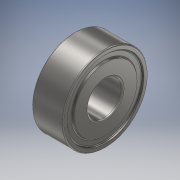
# Autodesk Inventor part: Rear Compression Bearing
Saved by Autodesk Inventor 2019 (Build 230136000, 136)
## iProperties
Created: 2017-03-14
Part Number: Rear Compression Bearing
Material: Stainless Steel
Document SubType Name: Modeling
Designer: zhangxun
Density: 8 g/cm^3
Appearance: Semi-Polished
Author: zhangxun
Autodesk Inventor part; units mm, degrees
ref_plane "YZ Plane" through (0, 0, 0) normal (1, 0, 0) x (0, 1, 0)
ref_plane "XZ Plane" through (0, 0, 0) normal (0, 1, 0) x (-1, 0, 0)
ref_plane "XY Plane" through (0, 0, 0) normal (0, 0, 1) x (1, 0, 0)
sketch "Sketch1" plane through (0, 0, 0) normal (0, 1, 0) x (-1, 0, 0)
  line L0 (19.5, 11) -> (1.5, 11)
  arc A0 (0.5, 12) -> (1.5, 11) centre (1.5, 12) ccw
  line L1 (0.5, 12) -> (0.5, 20.35)
  line L2 (0.5, 20.35) -> (2.3602, 20.35)
  arc A1 (1.5, 21.2102) -> (2.3602, 20.35) centre (2.3602, 21.2102) ccw
  line L3 (1.5, 21.2102) -> (1.5, 23.7908)
  arc A2 (2.3187, 24.65) -> (1.5, 23.7908) centre (2.3602, 23.7908) ccw
  line L4 (2.3187, 24.65) -> (1.5, 24.65)
  line L5 (1.5, 24.65) -> (1.5, 24.7964)
  line L6 (1.5, 24.7964) -> (0.5, 24.7964)
  line L7 (0.5, 24.7964) -> (0.5, 26.9)
  arc A3 (1.1, 27.5) -> (0.5, 26.9) centre (1.1, 26.9) ccw
  line L8 (1.1, 27.5) -> (19.9, 27.5)
  arc A4 (20.5, 26.9) -> (19.9, 27.5) centre (19.9, 26.9) ccw
  line L9 (20.5, 26.9) -> (20.5, 24.8239)
  line L10 (20.5, 24.8239) -> (19.5, 24.8239)
  line L11 (19.5, 24.8239) -> (19.5, 24.65)
  line L12 (19.5, 24.65) -> (18.6813, 24.65)
  arc A5 (19.5, 23.7908) -> (18.6813, 24.65) centre (18.6398, 23.7908) ccw
  line L13 (19.5, 23.7908) -> (19.5, 21.2102)
  arc A6 (18.6398, 20.35) -> (19.5, 21.2102) centre (18.6398, 21.2102) ccw
  line L14 (18.6398, 20.35) -> (20.5, 20.35)
  line L15 (20.5, 20.35) -> (20.5, 12)
  arc A7 (19.5, 11) -> (20.5, 12) centre (19.5, 12) ccw
  line L16 (0, 0) -> (63.5956, 0)
  dimension "d2" = 55
  dimension "d3" = 22
  dimension "d4" = 40.7
  dimension "d5" = 49.6479
  dimension "d6" = 49.5929
  constraints: 34 end point, 16 point on circle, 8 centre point, 1 horizontal
  measures "d2" diameter of L8 L16
  measures "d3" diameter of L0 L16
  measures "d4" diameter of L14 L16
  measures "d5" diameter of L10 L16
  measures "d6" diameter of L6 L16
revolve "Revolution1" add sketch "Sketch1" angle 360 about axis through (0, 0, 0) along (-1, 0, 0)
body "Solid2"
